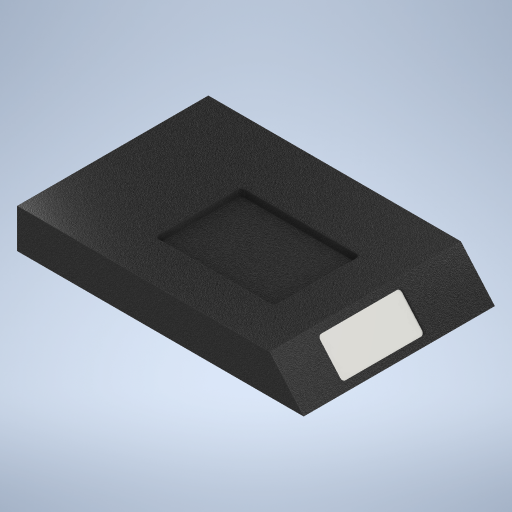
# Autodesk Inventor part: 3d
Saved by Autodesk Inventor 2023 (Build 270158000, 158)
## iProperties
Created: 2023-03-08
Part Number: 3d
Material: Типовые
Document SubType Name: Modeling
Designer: Josh
Density: 1 g/cm^3
Appearance: Черный — литой
Author: Josh
Autodesk Inventor part; units mm, degrees
ref_plane "YZ Plane" through (0, 0, 0) normal (1, 0, 0) x (0, 1, 0)
ref_plane "XZ Plane" through (0, 0, 0) normal (0, 1, 0) x (-1, 0, 0)
ref_plane "XY Plane" through (0, 0, 0) normal (0, 0, 1) x (1, 0, 0)
sketch "Эскиз1" plane through (0, 0, 0) normal (0, 1, 0) x (-1, 0, 0)
  line L0 (-67.75, -52) -> (67.75, -52)
  line L1 (71.75, -48) -> (71.75, 48)
  line L2 (67.75, 52) -> (-67.75, 52)
  line L3 (-71.75, 48) -> (-71.75, -48)
  line L4 (-71.75, -52) -> (71.75, 52) construction
  line L5 (71.75, -52) -> (-71.75, 52) construction
  arc A0 (71.75, 48) -> (67.75, 52) centre (67.75, 48) ccw
  arc A1 (67.75, -52) -> (71.75, -48) centre (67.75, -48) ccw
  arc A2 (-71.75, -48) -> (-67.75, -52) centre (-67.75, -48) ccw
  arc A3 (-67.75, 52) -> (-71.75, 48) centre (-67.75, 48) ccw
  line L6 (185.8649, 102) -> (-116.75, 102)
  line L7 (-116.75, 102) -> (-116.75, -127)
  line L8 (-116.75, -127) -> (185.8649, -127)
  line L9 (185.8649, -127) -> (185.8649, 102)
  point P0 (0, 0)
  point P1 (34.5574, -127)
  dimension "d0" = 143.5
  dimension "d1" = 104
  dimension "d2" = 4
  dimension "d3" = 45
  dimension "d4" = 50
  dimension "d5" = 75
  constraints: 20 end point, 8 point on circle, 8 point on line, 8 tangent, 4 centre point, 4 parallel, 3 equal radius, 3 midpoint, 2 horizontal, 2 perpendicular
  measures "d0" distance of L5.end L4.end
  measures "d1" distance of L4.end L5.start
  measures "d2" radius of A0
  measures "d3" distance between parallel lines of L7 L3
  measures "d4" distance between parallel lines of L2 L6
  measures "d5" distance from line of point (34.557, -127) L0
extrude "Выдавливание1" add sketch "Эскиз1" against normal blind 10
sketch "Эскиз2" plane through (-185.8649, 0, 102) normal (0, 0, 1) x (1, 0, 0)
  line L0 (0, 0) -> (302.6149, 0) projected
  line L1 (302.6149, 0) -> (343.2905, -46.792)
  line L2 (343.2905, -46.792) -> (0, -46.792)
  line L3 (0, 0) -> (0, -10) projected
  line L4 (0, -46.792) -> (0, 0)
  line L5 (0, 0) -> (302.6149, 0) projected
  line L6 (0, 0) -> (0, -10) projected
  line L7 (302.6149, -10) -> (0, -10) projected
  line L8 (302.6149, 0) -> (302.6149, -10) projected
  point P0 (185.8649, 0)
  point P1 (302.6149, 0)
  point P2 (0, -10)
  dimension "d8" = 131
  dimension "d9" = 62
  constraints: 6 end point, 1 horizontal, 1 perpendicular
  measures "d8" angle of L1 L0
  measures "d9" distance of L0.end L1.end
extrude "Выдавливание2" add sketch "Эскиз2" against normal up to surface (229 mm away) contours L1 L2 L4 L7 L8
sketch "Эскиз3" plane through (116.75, 0, 102) normal (0.7547, 0.6561, 0) x (0, 0, -1)
  line L0 (56, -8.5) -> (148, -8.5)
  line L1 (152, -12.5) -> (152, -49.5)
  line L2 (148, -53.5) -> (56, -53.5)
  line L3 (52, -49.5) -> (52, -12.5)
  line L4 (0, 0) -> (229, 0) projected
  line L5 (154, 121.0429) -> (154, 32.1469) projected
  arc A0 (56, -8.5) -> (52, -12.5) centre (56, -12.5) ccw
  arc A1 (152, -12.5) -> (148, -8.5) centre (148, -12.5) ccw
  arc A2 (148, -53.5) -> (152, -49.5) centre (148, -49.5) ccw
  arc A3 (52, -49.5) -> (56, -53.5) centre (56, -49.5) ccw
  line L6 (102, -8.5) -> (102, -53.5)
  line L7 (150, 29.5227) -> (54, 29.5227) projected
  point P0 (102, 76.5949)
  point P1 (102, 29.5227)
  dimension "d12" = 100
  dimension "d13" = 45
  dimension "d14" = 8.5
  dimension "d16" = 4
  constraints: 10 end point, 8 point on circle, 8 tangent, 4 centre point, 3 equal radius, 3 midpoint, 2 parallel, 1 horizontal, 1 perpendicular, 1 vertical alignment
  measures "d12" distance between parallel lines of L3 L1
  measures "d13" distance between parallel lines of L2 L0
  measures "d14" distance between parallel lines of L4 L0
  measures "d16" radius of A0
extrude "Выдавливание3" cut sketch "Эскиз3" against normal blind 2
